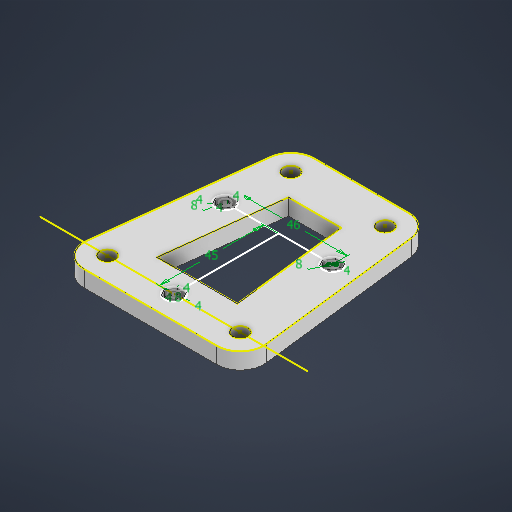
# Autodesk Inventor part: 라이다
Saved by Autodesk Inventor 2026.2 (Build 302298000, 298)
## iProperties
Created: 2025-11-27
Part Number: 라이다
Material: 일반
Document SubType Name: Modeling
Designer: PC
Density: 1 g/cm^3
Appearance: 기본값
Author: PC
Autodesk Inventor part; units mm, degrees
ref_plane "YZ Plane" through (0, 0, 0) normal (1, 0, 0) x (0, 1, 0)
ref_plane "XZ Plane" through (0, 0, 0) normal (0, 1, 0) x (-1, 0, 0)
ref_plane "XY Plane" through (0, 0, 0) normal (0, 0, 1) x (1, 0, 0)
sketch "스케치1" plane through (0, 0, 0) normal (0, 1, 0) x (-1, 0, 0)
  line L0 (28.5, 0) -> (-28.5, 0)
  line L1 (-26.25, 0) -> (-30.75, 0)
  circle A0 centre (-28.5, 0) radius 10
  line L2 (0, -98.6) -> (0, 28.1) projected
  line L3 (53.9, 0) -> (-53.9, 0) projected
  circle A1 centre (28.5, 0) radius 10
  line L4 (20.25, -70.5) -> (-20.25, -70.5)
  circle A2 centre (-20.25, -70.5) radius 10
  circle A3 centre (-20.25, -70.5) radius 3.25
  circle A4 centre (20.25, -70.5) radius 10
  line L5 (30.1822, -71.6623) -> (38.4322, -1.1623)
  line L6 (20.25, -80.5) -> (-20.25, -80.5)
  line L7 (28.5, 10) -> (-28.5, 10)
  line L8 (-30.1822, -71.6623) -> (-38.4322, -1.1623)
  line L9 (10.3178, -69.3377) -> (18.5678, 1.1623)
  line L10 (20.25, -60.5) -> (-20.25, -60.5)
  line L11 (-10.3178, -69.3377) -> (-18.5612, 1.1063)
  line L12 (27.5, -10) -> (-28.5, -10)
  circle A5 centre (-28.5, 0) radius 3.25
  circle A6 centre (20.25, -70.5) radius 3.25
  circle A7 centre (28.5, 0) radius 3.25
  point P0 (0, 0)
  point P1 (0, 0)
  point P2 (0, -70.5)
  point P3 (-17, -70.5)
  point P4 (-23.5, -70.5)
  point P5 (18.5, 0)
  point P6 (18.4318, 0)
  point P7 (-18.0599, 1.0927)
  point P8 (-18.4318, 0)
  point P9 (-18.5, 0)
  point P10 (-11.352, -60.5)
  point P11 (-17.2616, -10)
  point P12 (17.2616, -10)
  point P13 (11.352, -60.5)
  dimension "d0" = 57
  dimension "d7" = 20
  dimension "d10" = 40.5
  dimension "d11" = 70.5
  dimension "d12" = 20
  dimension "d13" = 6.5
  dimension "d17" = 6.5
  dimension "d18" = 6.5
  dimension "d19" = 6.5
  constraints: 22 end point, 12 point on circle, 11 tangent, 8 centre point, 7 coincident, 4 horizontal, 4 parallel, 3 midpoint, 2 point on line, 2 symmetric about line, 2 other
  measures "d0" distance of L0.end L0.start
  measures "d7" diameter of A0
  measures "d10" distance of L4.start L4.end
  measures "d11" distance between parallel lines of L4 L0
  measures "d12" diameter of A2
  measures "d13" diameter of A3
  measures "d17" diameter of A5
  measures "d18" diameter of A6
  measures "d19" diameter of A7
extrude "돌출1" add sketch "스케치1" along normal blind 7 contours A0 L3 A5 L0 | A0 L11 L0 | L0 A5 L3 A0 | L0 L11 L12 A0 | L11 A0 L7 L2 L0 | L0 L2 L12 L11 | L12 L11 L10 A2 L8 A0 | L2 L7 A1 L9 L0 | L0 L9 L12 L2 | L9 A1 L0 | L0 A1 L5 A4 L10 L9 | L11 A2 L10 | L10 L2 L4 A2 L11 | A2 | A1 L3 A7 L0 | L0 A7 L3 A1 | L10 L9 A4 L4 L2 | A2 L4 L2 L6 | L10 A4 L9 | L4 A4 L6 L2 | A4
sketch "스케치2" plane through (0, 7, 0) normal (0, 1, 0) x (1, 0, 0)
  point P0 (0, 0)
sketch "스케치3" plane through (0, 7, 0) normal (0, 1, 0) x (1, 0, 0)
  circle A0 centre (0, 0) radius 4
  line L0 (-30.1822, 71.6623) -> (-38.4322, 1.1623) projected
  arc A1 (-38.4322, 1.1623) -> (-28.5, -10) centre (-28.5, 0) ccw projected
  line L1 (-28.5, -10) -> (28.5, -10) projected
  arc A2 (28.5, -10) -> (38.4322, 1.1623) centre (28.5, 0) ccw projected
  line L2 (38.4322, 1.1623) -> (30.1822, 71.6623) projected
  arc A3 (30.1822, 71.6623) -> (20.25, 80.5) centre (20.25, 70.5) ccw projected
  line L3 (20.25, 80.5) -> (-20.25, 80.5) projected
  arc A4 (-20.25, 80.5) -> (-30.1822, 71.6623) centre (-20.25, 70.5) ccw projected
  circle A5 centre (20.25, 70.5) radius 3.25 projected
  line L4 (11.352, 60.5) -> (17.2616, 10) projected
  line L5 (17.2616, 10) -> (-17.2616, 10) projected
  line L6 (-17.2616, 10) -> (-11.352, 60.5) projected
  line L7 (-11.352, 60.5) -> (11.352, 60.5) projected
  circle A6 centre (28.5, 0) radius 3.25 projected
  circle A7 centre (-28.5, 0) radius 3.25 projected
  circle A8 centre (-20.25, 70.5) radius 3.25 projected
  line L8 (0, 0) -> (0, 45)
  line L9 (-23, 45) -> (23, 45)
  circle A9 centre (-23, 45) radius 4
  circle A10 centre (23, 45) radius 4
  line L10 (-2, 3.4641) -> (2, 3.4641)
  line L11 (-2, 3.4641) -> (-4, 0)
  line L12 (57.3115, 0) -> (-57.3115, 0) projected
  line L13 (-4, 0) -> (-2, -3.4641)
  line L14 (-2, -3.4641) -> (2, -3.4641)
  line L15 (4, 0) -> (2, -3.4641)
  line L16 (4, 0) -> (2, 3.4641)
  line L17 (-25, 48.4641) -> (-21, 48.4641)
  line L18 (-25, 48.4641) -> (-27, 45)
  line L19 (-21, 48.4641) -> (-19, 45)
  line L20 (-19, 45) -> (-21, 41.5359)
  line L21 (-25, 41.5359) -> (-21, 41.5359)
  line L22 (-25, 41.5359) -> (-27, 45)
  line L23 (25, 48.4641) -> (21, 48.4641)
  line L24 (25, 48.4641) -> (27, 45)
  line L25 (21, 48.4641) -> (19, 45)
  line L26 (19, 45) -> (21, 41.5359)
  line L27 (25, 41.5359) -> (21, 41.5359)
  line L28 (25, 41.5359) -> (27, 45)
  circle A11 centre (-23, 45) radius 2
  circle A12 centre (23, 45) radius 2
  circle A13 centre (0, 0) radius 2
  dimension "d20" = 8
  dimension "d21" = 45
  dimension "d22" = 46
  dimension "d23" = 8
  dimension "d24" = 8
  dimension "d25" = 4
  dimension "d26" = 4
  dimension "d27" = 4
  dimension "d28" = 4
  dimension "d31" = 4
  dimension "d32" = 4
  dimension "d33" = 4
  constraints: 40 end point, 6 coincident, 6 point on circle, 6 symmetric about line, 5 centre point, 4 parallel, 3 horizontal, 3 point on line, 1 midpoint, 1 perpendicular, 1 vertical, 9 other
  measures "d21" distance of L8.end L8.start
  measures "d22" distance of L9.start L9.end
  measures "d23" diameter of A9
  measures "d24" diameter of A10
  measures "d25" distance of L10.start L10.end
  measures "d26" distance of L13.end L14.end
  measures "d27" distance of L17.start L17.end
  measures "d28" distance of L21.start L20.end
  measures "d31" diameter of A11
  measures "d32" diameter of A13
  measures "d33" diameter of A12
extrude "돌출2" cut sketch "스케치3" against normal blind 3 contours L15 L14 L13 L12 A13 | A11 | L20 L21 L22 L18 L17 L19 | A12 | L25 L23 L24 L28 L27 L26 | L12 A13 L8 L10 L16 | A13 L12 | L12 L8 A13 | L8 A13 L12 L11 L10 | L12 A13 L8
extrude "돌출3" cut sketch "스케치3" against normal blind 7 contours A11 | A12 | A13 L12 | L12 L8 A13 | L12 A13 L8
